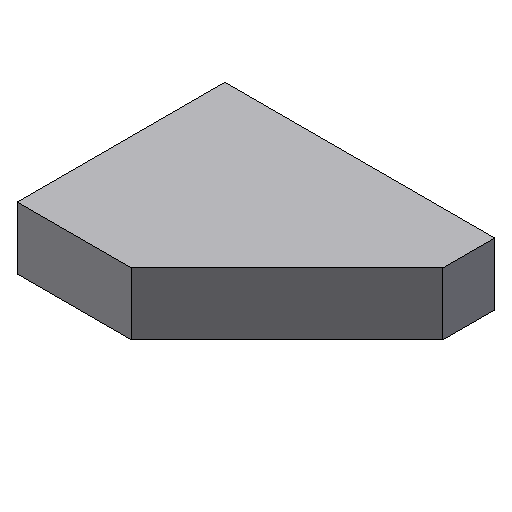
# Autodesk Inventor part: TL20240701-10110CV-003
Saved by Autodesk Inventor 2022.5 (Build 265521000, 521)
## iProperties
Category: DRIVE UNIT ASSY
Company: 현대 트랜시스(대유)
Created: 2023-05-17
Part Number: TL20240701-10110CV-003
Checked By: 김형민
Engr Approved By: 김시현
User Status: 8 x18
Material: SS400
Description: 0
Document SubType Name: Modeling
Mfg Approved By: 호상태
Designer: 김건휴
Stock Number: 003
Density: 7.85 g/cm^3
Appearance: Painting-RAL7035
Project: SW PJT
DETAIL: Coveryor Assembly
M/C TITLE: CJ 제일제당 협동로봇 포장시스탬 PILOT 장비
PARTS NAME: Bracket
SPECIFICATION: TA20221101-CV200000-015
DocNumber: 221118_Standard_v1
Folder: .\
VDS_Category: 엔지니어링
Detail Description: Processed products
Title: BLOCK
Subject: SW차종 시트조립라인
Author: 김건휴
Revision Number: A
Autodesk Inventor part; units mm, degrees
ref_plane "YZ Plane" through (0, 0, 0) normal (1, 0, 0) x (0, 1, 0)
ref_plane "XZ Plane" through (0, 0, 0) normal (0, 1, 0) x (-1, 0, 0)
ref_plane "XY Plane" through (0, 0, 0) normal (0, 0, 1) x (1, 0, 0)
sketch "스케치9" plane through (0, 0, 0) normal (0, 1, 0) x (-1, 0, 0)
  line L0 (-26, 20) -> (26, 20)
  line L1 (26, 20) -> (26, -20)
  line L2 (26, -20) -> (-26, -20)
  line L3 (-26, -20) -> (-26, 20)
  line L4 (-26, 20) -> (26, -20) construction
  line L5 (26, 20) -> (-26, -20) construction
  line L6 (4, 20) -> (-26, -10)
  point P0 (0, 0)
  dimension "d40" = 52
  dimension "d41" = 40
  dimension "d42" = 30
  dimension "d43" = 10
  constraints: 14 end point, 2 midpoint, 2 parallel, 2 point on line, 1 horizontal, 1 perpendicular
  measures "d40" distance of L0.start L0.end
  measures "d41" distance of L0.end L1.end
  measures "d42" distance of L0.start L6.start
  measures "d43" distance of L2.end L6.end
extrude "돌출4" add sketch "스케치9" along normal mid plane 12 contours L0 L1 L2 L3 L6
sketch "스케치10" plane through (26, 6, -20) normal (0, 0, -1) x (-1, 0, 0)
  line L0 (0, -12) -> (0, 0) projected
  point P0 (26, -6)
  point P1 (8, -6)
  point P2 (23, -6)
  dimension "d47" = 15
  dimension "d48" = 8
  constraints: 2 horizontal alignment
  measures "d47" distance of point (23, -6) point (8, -6)
  measures "d48" distance from line of L0 point (8, -6)
hole "구멍3" at (18, 0, -20) at (3, 0, -20) direction (0, 0, 1) diameter 4.917 depth 12 tip angle 118 thread size "M6x1" class "6H" standard "ISO Metric profile"
sketch "스케치11" plane through (-26, -6, 20) normal (-1, 0, 0) x (0, 0, 1)
  line L0 (0, 0) -> (0, 12) projected
  line L1 (-40, 12) -> (0, 12) projected
  point P0 (-20, 6)
  point P1 (-23, 6)
  point P2 (-8, 6)
  point P3 (0, 6)
  dimension "d56" = 15
  dimension "d57" = 8
  dimension "d58" = 6
  constraints: 1 horizontal alignment, 1 midpoint
  measures "d56" distance of point (-23, 6) point (-8, 6)
  measures "d57" distance of point (0, 6) point (-8, 6)
  measures "d58" distance from line of L1 point (-8, 6)
hole "구멍4" at (-26, 0, -3) at (-26, 0, 12) direction (1, 0, 0) diameter 4.917 depth 12 tip angle 118 thread size "M6x1" class "6H" standard "ISO Metric profile"
